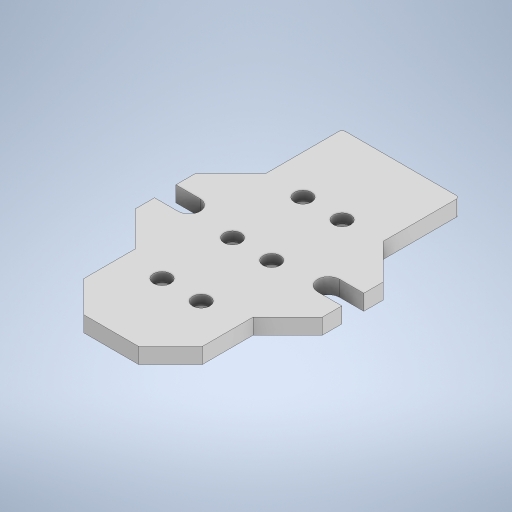
# Autodesk Inventor part: Groundplate
Saved by Autodesk Inventor 2023 (Build 270158000, 158)
## iProperties
Created: 2023-05-10
Part Number: Groundplate
Material: Generic
Document SubType Name: Modeling
Designer: dell
Density: 1 g/cm^3
Appearance: Default
Author: dell
Autodesk Inventor part; units mm, degrees
ref_plane "YZ Plane" through (0, 0, 0) normal (1, 0, 0) x (0, 1, 0)
ref_plane "XZ Plane" through (0, 0, 0) normal (0, 1, 0) x (-1, 0, 0)
ref_plane "XY Plane" through (0, 0, 0) normal (0, 0, 1) x (1, 0, 0)
sketch "Sketch1" plane through (0, 0, 0) normal (0, 1, 0) x (-1, 0, 0)
  arc A0 (-44.5, -7) -> (-44.5, 7) centre (-44.5, 0) ccw
  arc A1 (44.5, 7) -> (44.5, -7) centre (44.5, 0) ccw
  line L0 (44.5, 7) -> (59.6236, 7)
  line L1 (44.5, -7) -> (60, -7)
  line L2 (-44.5, 7) -> (-60, 7)
  line L3 (-44.5, -7) -> (-60, -7)
  line L4 (60, -7) -> (60, -19.5)
  line L5 (-60, 7) -> (-60, 19.5)
  line L6 (59.6236, 7) -> (59.6236, 19.5)
  line L7 (-60, -7) -> (-60, -19.5)
  line L8 (37.5, -90.6623) -> (-37.5, -90.6623)
  line L9 (17.5, 94.3377) -> (-17.5, 94.3377)
  line L10 (60, -19.5) -> (37.5, -42)
  line L11 (-60, -19.5) -> (-37.5, -42)
  line L12 (37.5, -90.6623) -> (37.5, -42)
  line L13 (-37.5, -90.6623) -> (-37.5, -42)
  line L14 (59.6236, 19.5) -> (37.5, 41.6236)
  line L15 (-60, 19.5) -> (-37.8764, 41.6236)
  line L16 (37.5, 41.6236) -> (37.5, 74.3377)
  line L17 (-37.8764, 41.6236) -> (-37.8764, 73.9613)
  line L18 (17.5, 94.3377) -> (37.5, 74.3377)
  line L19 (-17.5, 94.3377) -> (-37.8764, 73.9613)
  point P0 (0, 0)
  dimension "d0" = 89
  dimension "d1" = 44.5
  dimension "d5" = 60
  dimension "d10" = 39
  dimension "d11" = 19.5
  dimension "d12" = 19.5
  dimension "d13" = 39
  dimension "d14" = 19.5
  dimension "d15" = 19.5
  dimension "d16" = 75
  dimension "d17" = 37.5
  dimension "d18" = 35
  dimension "d19" = 17.5
  dimension "d20" = 185
  dimension "d22" = 45
  dimension "d23" = 45
  dimension "d24" = 45
  dimension "d25" = 45
  dimension "d28" = 45
  dimension "d29" = 45
  constraints: 40 end point, 7 vertical, 6 horizontal, 4 point on circle, 4 tangent, 2 centre point, 1 point on line
  measures "d0" distance of A0.centre A1.centre
  measures "d1" distance of point (0, 0) A0.centre
  measures "d5" distance from line of point (0, 0) L4
  measures "d10" distance of L5.end L7.end
  measures "d11" vertical distance of A0.centre L7.end
  measures "d12" vertical distance of L5.end A0.centre
  measures "d13" vertical distance of L6.end L4.end
  measures "d14" vertical distance of A1.centre L6.end
  measures "d15" vertical distance of A1.centre L4.end
  measures "d16" distance of L8.start L8.end
  measures "d17" horizontal distance of point (0, 0) L8.end
  measures "d18" distance of L9.start L9.end
  measures "d19" horizontal distance of point (0, 0) L9.end
  measures "d20" distance between parallel lines of L9 L8
  measures "d22" angle of L4 L10
  measures "d23" angle of L7 L11
  measures "d24" angle of L6 L14
  measures "d25" angle of L5 L15
  measures "d28" angle of L17 L19
  measures "d29" angle of L16 L18
extrude "Extrusion1" add sketch "Sketch1" along normal blind 10
sketch "Sketch2" plane through (0, 10, 0) normal (0, 1, 0) x (1, 0, 0)
  circle A0 centre (-12.5, 40.6623) radius 5.5
  circle A1 centre (-12.5, -4.3377) radius 5.5
  circle A2 centre (-12.5, -49.3377) radius 5.5
  line L0 (37.5, 90.6623) -> (-37.5, 90.6623) projected
  circle A3 centre (12.5, -49.3377) radius 5.5
  circle A4 centre (12.5, -4.3377) radius 5.5
  circle A5 centre (12.5, 40.6623) radius 5.5
  point P0 (0, 0)
  dimension "d32" = 11
  dimension "d33" = 11
  dimension "d34" = 11
  dimension "d35" = 50
  dimension "d36" = 45
  dimension "d37" = 45
  dimension "d38" = 11
  dimension "d39" = 11
  dimension "d40" = 11
  dimension "d41" = 25
  dimension "d42" = 12.5
  dimension "d43" = 12.5
  dimension "d44" = 12.5
  dimension "d45" = 12.5
  dimension "d46" = 12.5
  constraints: 6 centre point
  measures "d32" diameter of A0
  measures "d33" diameter of A1
  measures "d34" diameter of A2
  measures "d35" distance from line of A0.centre L0
  measures "d36" distance of A1.centre A0.centre
  measures "d37" distance of A2.centre A1.centre
  measures "d38" diameter of A5
  measures "d39" diameter of A4
  measures "d40" diameter of A3
  measures "d41" distance of A0.centre A5.centre
  measures "d42" horizontal distance of point (0, 0) A0.centre
  measures "d43" horizontal distance of point (0, 0) A4.centre
  measures "d44" horizontal distance of point (0, 0) A3.centre
  measures "d45" horizontal distance of point (0, 0) A1.centre
  measures "d46" horizontal distance of point (0, 0) A5.centre
extrude "Extrusion2" cut sketch "Sketch2" against normal blind 6
sketch "Sketch3" plane through (-12.5, 4, 4.3377) normal (0, 1, 0) x (1, 0, 0)
  circle A0 centre (0, 0) radius 3
  circle A1 centre (25, 0) radius 5.5 projected
  circle A2 centre (25, 0) radius 3
  circle A3 centre (0, -45) radius 5.5 projected
  circle A4 centre (0, -45) radius 3
  circle A5 centre (0, 45) radius 5.5 projected
  circle A6 centre (25, 45) radius 5.5 projected
  circle A7 centre (25, -45) radius 3
  circle A8 centre (25, 45) radius 3
  circle A9 centre (0, 45) radius 3
  point P0 (12.5, 4.3377)
  dimension "d51" = 6
  dimension "d52" = 6
  dimension "d53" = 6
  dimension "d55" = 6
  dimension "d56" = 6
  dimension "d57" = 6
  constraints: 7 coincident, 6 centre point
  measures "d51" diameter of A0
  measures "d52" diameter of A2
  measures "d53" diameter of A4
  measures "d55" diameter of A9
  measures "d56" diameter of A8
  measures "d57" diameter of A7
extrude "Extrusion3" cut sketch "Sketch3" against normal blind 6 contours A0 | A2 | A4 | A7 | A8 | A9
fillet "Fillet1" radius 2 1 edges at (-37.5, 5, -90.6623)
fillet "Fillet2" radius 2 1 edges at (37.5, 5, -90.6623)
body "Solid1"
